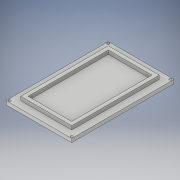
# Autodesk Inventor part: mien_top
Saved by Autodesk Inventor 2019 (Build 230136000, 136)
## iProperties
Created: 2018-11-23
Part Number: mien_top
Material: Generic
Document SubType Name: Modeling
Designer: jerem
Density: 1 g/cm^3
Appearance: Default
Author: jerem
Autodesk Inventor part; units mm, degrees
ref_plane "YZ Plane" through (0, 0, 0) normal (1, 0, 0) x (0, 1, 0)
ref_plane "XZ Plane" through (0, 0, 0) normal (0, 1, 0) x (-1, 0, 0)
ref_plane "XY Plane" through (0, 0, 0) normal (0, 0, 1) x (1, 0, 0)
sketch "Sketch1" plane through (0, 0, 0) normal (0, 1, 0) x (-1, 0, 0)
  line L0 (62.65, 0) -> (-62.65, 0) projected
  line L1 (0, -97.65) -> (0, 97.65) projected
  line L2 (44.75, -69.75) -> (-44.75, -69.75)
  line L3 (-44.75, -69.75) -> (-44.75, 69.75)
  line L4 (-44.75, 69.75) -> (44.75, 69.75)
  line L5 (44.75, 69.75) -> (44.75, -69.75)
  point P0 (0, 0)
  dimension "d0" = 89.5
  dimension "d1" = 139.5
  dimension "d2" = 69.75
  dimension "d3" = 44.75
  constraints: 8 end point, 2 parallel, 1 horizontal, 1 perpendicular
  measures "d0" distance of L3.end L4.end
  measures "d1" distance of L2.end L3.end
  measures "d2" distance between parallel lines of L4 L0
  measures "d3" distance between parallel lines of L1 L3
extrude "Extrusion1" add sketch "Sketch1" along normal blind 5
sketch "Sketch2" plane through (0, 5, 0) normal (0, 1, 0) x (1, 0, 0)
  circle A0 centre (-42.375, 67.375) radius 1.625
  circle A1 centre (42.375, 67.375) radius 1.625
  circle A2 centre (42.375, -67.375) radius 1.625
  circle A3 centre (-42.375, -67.375) radius 1.625
  line L0 (44.75, -69.75) -> (44.75, 69.75) projected
  line L1 (44.75, 69.75) -> (-44.75, 69.75) projected
  line L2 (-44.75, 69.75) -> (-44.75, -69.75) projected
  line L3 (-44.75, -69.75) -> (44.75, -69.75) projected
  dimension "d6" = 3.25
  dimension "d9" = 3.25
  dimension "d12" = 3.25
  dimension "d15" = 3.25
  dimension "d19" = 2.375
  dimension "d20" = 2.375
  dimension "d21" = 2.375
  dimension "d22" = 2.375
  dimension "d23" = 2.375
  dimension "d24" = 2.375
  dimension "d25" = 2.375
  dimension "d26" = 2.375
  constraints: 4 centre point
  measures "d6" diameter of A0
  measures "d9" diameter of A1
  measures "d12" diameter of A2
  measures "d15" diameter of A3
  measures "d19" distance from line of L0 A1.centre
  measures "d20" distance from line of L1 A1.centre
  measures "d21" distance from line of L2 A0.centre
  measures "d22" distance from line of L1 A0.centre
  measures "d23" distance from line of L3 A3.centre
  measures "d24" distance from line of L2 A3.centre
  measures "d25" distance from line of L0 A2.centre
  measures "d26" distance from line of L3 A2.centre
extrude "Extrusion2" cut sketch "Sketch2" against normal blind 5 contours A0 | A1 | A2 | A3
sketch "Sketch3" plane through (0, 5, 0) normal (0, 1, 0) x (1, 0, 0)
  line L0 (-34.75, -59.75) -> (34.75, -59.75)
  line L1 (34.75, -59.75) -> (34.75, 59.75)
  line L2 (34.75, 59.75) -> (-34.75, 59.75)
  line L3 (-34.75, 59.75) -> (-34.75, -59.75)
  circle A0 centre (42.375, -67.375) radius 1.625 projected
  circle A1 centre (-42.375, 67.375) radius 1.625 projected
  circle A2 centre (42.375, 67.375) radius 1.625 projected
  circle A3 centre (-42.375, -67.375) radius 1.625 projected
  line L4 (44.75, 69.75) -> (-44.75, 69.75) projected
  line L5 (-44.75, 69.75) -> (-44.75, -69.75) projected
  line L6 (-44.75, -69.75) -> (44.75, -69.75) projected
  line L7 (44.75, -69.75) -> (44.75, 69.75) projected
  line L8 (-29.75, 54.75) -> (29.75, 54.75)
  line L9 (29.75, 54.75) -> (29.75, -54.75)
  line L10 (29.75, -54.75) -> (-29.75, -54.75)
  line L11 (-29.75, -54.75) -> (-29.75, 54.75)
  point P0 (0, 0)
  dimension "d29" = 10
  dimension "d30" = 10
  dimension "d31" = 10
  dimension "d32" = 10
  dimension "d33" = 5
  dimension "d34" = 5
  dimension "d35" = 5
  dimension "d36" = 5
  constraints: 16 end point, 4 parallel, 2 horizontal, 2 perpendicular
  measures "d29" distance between parallel lines of L7 L1
  measures "d30" distance between parallel lines of L4 L2
  measures "d31" distance between parallel lines of L5 L3
  measures "d32" distance between parallel lines of L6 L0
  measures "d33" distance between parallel lines of L2 L8
  measures "d34" distance between parallel lines of L1 L9
  measures "d35" distance between parallel lines of L0 L10
  measures "d36" distance between parallel lines of L3 L11
extrude "Extrusion3" add sketch "Sketch3" along normal blind 5 contours L3 L2 L1 L0
body "Solid1"
